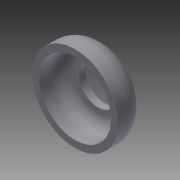
# Autodesk Inventor part: BallBearingCup
Saved by Autodesk Inventor 2015 (Build 190159000, 159)
## iProperties
Created: 2017-01-13
Part Number: BallBearingCup
Material: Generic
Document SubType Name: Modeling
Designer: 1esh9
Density: 1 g/cm^3
Appearance: Default
Author: 1esh9
Autodesk Inventor part; units mm, degrees
ref_plane "YZ Plane" through (0, 0, 0) normal (1, 0, 0) x (0, 1, 0)
ref_plane "XZ Plane" through (0, 0, 0) normal (0, 1, 0) x (-1, 0, 0)
ref_plane "XY Plane" through (0, 0, 0) normal (0, 0, 1) x (1, 0, 0)
sketch "Sketch1" plane through (0, 0, 0) normal (0, 0, 1) x (1, 0, 0)
  line L0 (0, 0) -> (5.5, 0) construction
  line L1 (5.5, 0) -> (5.5, -2)
  line L2 (0, -8.6) -> (12.34, -8.6) construction
  line L3 (12.34, -8.6) -> (12.34, -5.5)
  line L4 (5.5, -2) -> (6.84, -2)
  line L5 (10.34, -5.5) -> (10.34, -8.6)
  line L6 (5.5, 0) -> (6.84, 0)
  arc A0 (10.34, -5.5) -> (6.84, -2) centre (6.84, -5.5) ccw
  arc A1 (12.34, -5.5) -> (6.84, 0) centre (6.84, -5.5) ccw
  line L7 (10.34, -8.6) -> (12.34, -8.6)
  line L8 (0, 0) -> (0, -8.6)
  dimension "d0" = 5.5
  dimension "d1" = 2
  dimension "d2" = 12.34
  dimension "d3" = 8.6
  dimension "d6" = 2
  dimension "d7" = 0
  dimension "d8" = 3.5
  dimension "d9" = 5.5
  constraints: 18 end point, 5 horizontal, 4 point on circle, 2 centre point, 2 tangent, 2 vertical, 1 perpendicular, 1 point on line
  measures "d0" distance of L0.start L0.end
  measures "d1" distance of L0.end L1.end
  measures "d2" distance of L2.start L2.end
  measures "d3" distance from line of L2 L0.start
  measures "d6" distance between parallel lines of L5 L3
  measures "d7" horizontal distance of L0.start L2.start
  measures "d8" radius of A0
  measures "d9" radius of A1
revolve "Revolution1" add sketch "Sketch1" angle 360 about axis through (0, 0, 0) along (0, -1, 0)
body "Solid1"
